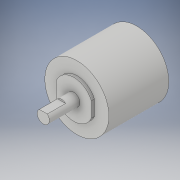
# Autodesk Inventor part: nhk_purry
Saved by Autodesk Inventor 2019 (Build 230136000, 136)
## iProperties
Created: 2022-02-27
Part Number: nhk_purry
Material: 一般
Document SubType Name: Sheet Metal
Designer: yuta
Density: 1 g/cm^3
Sheet Metal Rule: Default_mm
Appearance: 既定
Author: yuta
Autodesk Inventor part; units mm, degrees
ref_plane "YZ Plane" through (0, 0, 0) normal (1, 0, 0) x (0, 1, 0)
ref_plane "XZ Plane" through (0, 0, 0) normal (0, 1, 0) x (-1, 0, 0)
ref_plane "XY Plane" through (0, 0, 0) normal (0, 0, 1) x (1, 0, 0)
sketch "スケッチ1" plane through (0, 0, 0) normal (0, 0, 1) x (1, 0, 0)
  circle A0 centre (0, 0) radius 21
  dimension "d0" = 42
  constraints: 1 centre point, 1 coincident
  measures "d0" diameter of A0
extrude "押し出し1" add sketch "スケッチ1" along normal blind 39.2
sketch "スケッチ2" plane through (0, 0, 39.2) normal (0, 0, 1) x (1, 0, 0)
  circle A0 centre (0, 0) radius 12.5
  dimension "d3" = 25
  constraints: 1 centre point, 1 coincident
  measures "d3" diameter of A0
extrude "押し出し2" add sketch "スケッチ2" along normal blind 2
sketch "スケッチ3" plane through (0, 0, 41.2) normal (0, 0, 1) x (1, 0, 0)
  circle A0 centre (0, 0) radius 4
  dimension "d6" = 8
  constraints: 1 centre point, 1 coincident
  measures "d6" diameter of A0
extrude "押し出し3" add sketch "スケッチ3" along normal blind 20
sketch "スケッチ4" plane through (0, 0, 61.2) normal (0, 0, 1) x (1, 0, 0)
  circle A0 centre (0, 0) radius 4 projected
  circle A1 centre (0, 0) radius 4 projected
  line L0 (-2.6458, 3) -> (2.6458, 3)
  point P0 (0, 3)
  dimension "d9" = 3
  constraints: 2 end point, 2 point on circle, 1 horizontal
  measures "d9" distance of A0.centre point (0, 3)
extrude "押し出し4" cut sketch "スケッチ4" against normal blind 12 contours L0 A0 picked at (-0.6179, 3.1815)
sketch "スケッチ5" plane through (0, 0, 41.2) normal (0, 0, 1) x (1, 0, 0)
  circle A0 centre (0, 0) radius 12.5 projected
  line L0 (-11.5, 4.899) -> (-11.5, -4.899)
  line L1 (11.5, -4.899) -> (11.5, 4.899)
  point P0 (-11.5, 0)
  point P1 (11.5, 0)
  dimension "d12" = 11.5
  dimension "d13" = 11.5
  constraints: 4 end point, 4 point on circle, 1 parallel, 1 vertical
  measures "d12" distance of point (-11.5, 0) A0.centre
  measures "d13" distance of A0.centre point (11.5, 0)
extrude "押し出し5" cut sketch "スケッチ5" against normal blind 2 contours A0 L1 | L0 A0
equation "\"BendRadius\" = Thickness"
equation "\"BendReliefWidth\" = Thickness"
equation "\"BendReliefDepth\" = 0.5 * Thickness"
equation "\"CornerReliefSize\" = 4 * Thickness"
equation "\"MinimumRemnant\" = 2 * Thickness"
equation "\"TransitionRadius\" = BendRadius"
equation "\"JacobiRadiusSize\" = BendRadius"
equation "\"GapSize\" = Thickness"
equation "\"Thickness\" = 0.5"
